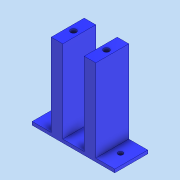
# Autodesk Inventor part: ir_sensor_support
Saved by Autodesk Inventor 2022 (Build 260153000, 153)
## iProperties
Created: 2021-09-16
Part Number: ir_sensor_support
Material: Generic
Document SubType Name: Modeling
Designer: nnico
Density: 1 g/cm^3
Appearance: Blue - Wall Paint - Glossy
Author: nnico
Autodesk Inventor part; units mm, degrees
ref_plane "YZ Plane" through (0, 0, 0) normal (1, 0, 0) x (0, 1, 0)
ref_plane "XZ Plane" through (0, 0, 0) normal (0, 1, 0) x (-1, 0, 0)
ref_plane "XY Plane" through (0, 0, 0) normal (0, 0, 1) x (1, 0, 0)
sketch "Sketch1" plane through (0, 0, 0) normal (0, 1, 0) x (-1, 0, 0)
  line L0 (-25, -10) -> (25, -10)
  line L1 (25, -10) -> (25, 10)
  line L2 (25, 10) -> (-25, 10)
  line L3 (-25, 10) -> (-25, -10)
  line L4 (-25, 0) -> (25, 0) construction
  line L5 (0, -10) -> (0, 10) construction
  point P0 (0, 0)
  point P1 (0, 0)
  dimension "d0" = 50
  dimension "d1" = 20
  constraints: 12 end point, 5 midpoint, 2 parallel, 1 coincident, 1 horizontal, 1 perpendicular
  measures "d0" distance of L2.end L1.end
  measures "d1" distance of L1.end L0.end
extrude "Extrusion1" add sketch "Sketch1" along normal blind 2
sketch "Sketch2" plane through (0, 2, 0) normal (0, 1, 0) x (1, 0, 0)
  line L0 (25, -10) -> (25, 10) construction
  line L1 (25, 0) -> (-30.0792, 0) construction
  line L2 (25, 10) -> (-25, 10) construction
  line L3 (0, 10) -> (0, -10) construction
  line L4 (-25, -10) -> (25, -10) construction
  circle A0 centre (18.5, 0) radius 1.5
  circle A1 centre (-18.5, 0) radius 1.5
  point P0 (0, 0)
  dimension "d4" = 3
  dimension "d5" = 37
  constraints: 4 end point, 3 midpoint, 2 centre point, 1 horizontal, 1 point on line, 1 symmetric about line, 1 other
  measures "d4" diameter of A0
  measures "d5" diameter of A0.centre L3
extrude "Extrusion2" cut sketch "Sketch2" against normal blind 2
sketch "Sketch6" plane through (0, 2, 0) normal (0, 1, 0) x (1, 0, 0)
  line L0 (25, 10) -> (-25, 10) construction
  line L1 (0, 10) -> (0, -10) construction
  line L2 (-25, -10) -> (25, -10) construction
  line L3 (6.5, 10) -> (13.5, 10)
  line L4 (13.5, 10) -> (13.5, -10)
  line L5 (13.5, -10) -> (6.5, -10)
  line L6 (6.5, -10) -> (6.5, 10)
  line L7 (-6.5, 10) -> (-13.5, 10)
  line L8 (-13.5, 10) -> (-13.5, -10)
  line L9 (-13.5, -10) -> (-6.5, -10)
  line L10 (-6.5, -10) -> (-6.5, 10)
  point P0 (0, 0)
  dimension "d19" = 7
  dimension "d20" = 6.5
  constraints: 18 end point, 4 symmetric about line, 2 midpoint, 2 parallel, 2 point on line, 1 horizontal, 1 perpendicular
  measures "d19" distance of L4.end L5.end
  measures "d20" distance of L3.start L1.start
extrude "Extrusion5" add sketch "Sketch6" along normal blind 50
sketch "Sketch7" plane through (0, 52, 0) normal (0, 1, 0) x (1, 0, 0)
  line L0 (6.5, 10) -> (-6.5, 10) construction
  line L1 (0, 10) -> (0, -10) construction
  line L2 (-6.5, -10) -> (6.5, -10) construction
  circle A0 centre (10, 0) radius 1.75
  line L3 (13.5, -10) -> (13.5, 10) construction
  circle A1 centre (-10, 0) radius 1.75
  point P0 (0, 0)
  dimension "d23" = 3.5
  dimension "d24" = 3.5
  constraints: 2 centre point, 2 end point, 2 midpoint, 1 symmetric about line, 1 other
  measures "d23" diameter of A0
  measures "d24" distance from line of L3 A0.centre
extrude "Extrusion6" cut sketch "Sketch7" against normal blind 6
body "Solid1"
